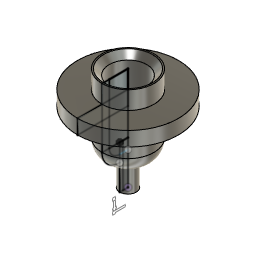
PNP Nozzle CP40 v17 (Autodesk Fusion 360 design; units mm, degrees)
Autodesk Fusion 360 part; units mm, degrees
sketch "Nozzle side view" plane through (0, 0, 0) normal (1, 0, 0) x (0, 1, 0)
  line L0 (0, 0) -> (-1.15, 0)
  line L1 (-1.15, 0) -> (-1.15, 6)
  line L2 (-1.15, 6) -> (0, 6)
  line L3 (0, 6) -> (0, 0)
  line L4 (0, 6) -> (-3.6, 6)
  line L5 (-3.6, 6) -> (-3.6, 14.3)
  line L6 (-3.6, 14.3) -> (0, 14.3)
  line L7 (0, 14.3) -> (0, 6)
  line L8 (0, 14.3) -> (0, 11.8) construction
  line L9 (0, 11.8) -> (-7, 11.8)
  line L10 (-7, 11.8) -> (-7, 9.8)
  line L11 (-7, 9.8) -> (0, 9.8)
  line L12 (0, 9.8) -> (0, 11.8)
  line L13 (0, 0) -> (-0.7, 0)
  line L14 (-0.7, 0) -> (-0.7, 6)
  line L15 (-0.7, 6) -> (0, 6)
  line L16 (0, 6) -> (0, 0)
  line L17 (0, 6) -> (-2.6, 6)
  line L18 (-2.6, 6) -> (-2.6, 14.3)
  line L19 (-2.6, 14.3) -> (0, 14.3)
  line L20 (0, 14.3) -> (0, 6)
  arc A0 (-2.6, 6) -> (-1.15, 4.55) centre (-1.15, 6) ccw
  arc A1 (-3.6, 6) -> (-1.15, 3.55) centre (-1.15, 6) ccw
  line L21 (-1.15, 4.55) -> (0, 4.55)
  dimension "d9" = 1.15
  dimension "d10" = 6
  dimension "d11" = 3.6
  dimension "d12" = 8.3
  dimension "d13" = 2.5
  dimension "d15" = 7
  dimension "d16" = 2
  dimension "d18" = 0.7
  dimension "d19" = 6
  dimension "d20" = 2.6
  dimension "d21" = 8.3
  dimension "d23" = 1.15
  constraint horizontal L0
  constraint vertical L1
  constraint horizontal L2
  constraint vertical L3
  constraint coincident L0.start L3.end
  constraint horizontal L4
  constraint vertical L5
  constraint horizontal L6
  constraint vertical L7
  constraint perpendicular L6 L8
  constraint horizontal L9
  constraint vertical L10
  constraint horizontal L11
  constraint vertical L12
  constraint horizontal L13
  constraint vertical L14
  constraint horizontal L15
  constraint vertical L16
  constraint horizontal L17
  constraint vertical L18
  constraint horizontal L19
  constraint vertical L20
  constraint coincident L1.end L2.start
  constraint horizontal L21
  measures "d9" distance of L0.start L0.end
  measures "d10" distance of L0.start L2.end
  measures "d11" distance of L2.end L4.end
  measures "d12" distance of L2.end L6.end
  measures "d13" distance of L6.end L8.end
  measures "d15" distance of L8.end L9.end
  measures "d16" distance of L8.end L11.end
  measures "d18" distance of L0.start L13.end
  measures "d19" distance of L0.start L2.end
  measures "d20" distance of L2.end L17.end
  measures "d21" distance of L2.end L6.end
  measures "d23" distance of A0.end L21.end
revolve "Revolve3" add sketch "Nozzle side view" angle 360 about axis through (0, 0, 6) along (0, 0, -1) contours L0 L1 L14 L21 | L1 L4 A0 A1 | L4 L5 L11 L18 | L5 L9 L11 L18 | L5 L9 L10 L11 | L5 L6 L9 L18
chamfer "Chamfer1" distance 0.8 angle 45 1 edges at (-2.4241, -0.9402, 14.3)
equation "id_nozzle_top = 5.2 mm" comment "inner diameter of the hole that accepts the metal motor shaft stock: 5.2"
equation "od_nozzle_top = id_nozzle_top + 2 mm" comment "outer diameter of the hole that accepts the metal motor shaft stock: 6.1"
equation "d_ring_for_toolchange = 14 mm" comment "diameter of the large ring around the nozzle for a toolchange stock: 10.4"
equation "l_upper_portion = 8.3 mm" comment "length / height of the thicker part of the nozzle stock: 8.3"
equation "id_nozzle_bottom = 0.7 mm" comment "stock: 0.7"
equation "od_nozzle_bottom = id_nozzle_bottom + 1.6 mm" comment "stock: 1.4"
equation "l_lower_portion = 6 mm" comment "stock: 6"
equation "dist_changing_ring_from_top = 2.5 mm" comment "stock: 2.5"
equation "d9 = od_nozzle_bottom / 2"
equation "d10 = l_lower_portion"
equation "d11 = od_nozzle_top / 2"
equation "d12 = l_upper_portion"
equation "d13 = dist_changing_ring_from_top"
equation "thickness_changing_ring = 2 mm" comment "stock: 1"
equation "d15 = d_ring_for_toolchange / 2"
equation "d16 = thickness_changing_ring"
equation "d18 = id_nozzle_bottom"
equation "d19 = l_lower_portion"
equation "d20 = id_nozzle_top / 2"
equation "d21 = l_upper_portion"
equation "d23 = od_nozzle_bottom / 2"
equation "d25 = ( od_nozzle_top - id_nozzle_top ) / 2 - 0.2 mm"
named bodies: "mm inner diameter Nozzle"
